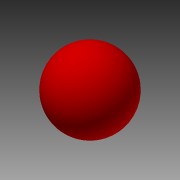
# Autodesk Inventor part: ball
Saved by Autodesk Inventor 2014 (Build 180170000, 170)
## iProperties
Created: 2014-01-12
Part Number: ball
Material: Ball material
Document SubType Name: Modeling
Designer: Tristan Debrunner
Density: 0.0114724 g/cm^3
Appearance: Generic
Author: Tristan Debrunner
Autodesk Inventor part; units mm, degrees
ref_plane "YZ Plane" through (0, 0, 0) normal (1, 0, 0) x (0, 1, 0)
ref_plane "XZ Plane" through (0, 0, 0) normal (0, 1, 0) x (-1, 0, 0)
ref_plane "XY Plane" through (0, 0, 0) normal (0, 0, 1) x (1, 0, 0)
sketch "Sketch1" plane through (0, 0, 0) normal (0, 0, 1) x (1, 0, 0)
  circle A0 centre (0, 0) radius 304.8
  line L0 (304.7962, -1.524) -> (-304.7962, 1.524)
  dimension "d0" = 609.6
  constraints: 2 end point, 2 point on circle, 1 centre point, 1 coincident, 1 midpoint
  measures "d0" diameter of A0
revolve "Revolution1" add sketch "Sketch1" angle 360 about axis through (304.7962, -1.524, 0) along (-0.9999875, 0.0049999, 0) picked at (-48.3498, 174.1022) contours A0 L0
body "Solid1"
